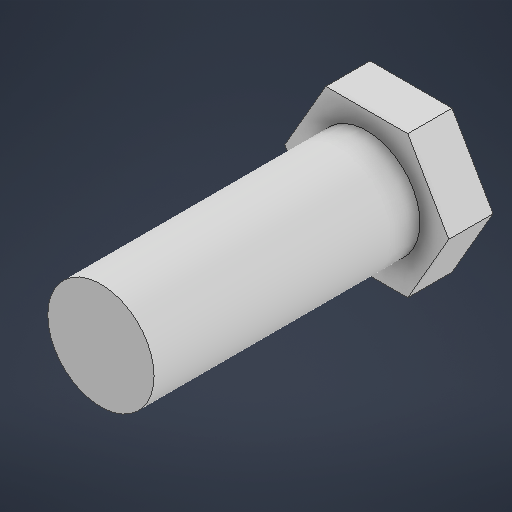
# Autodesk Inventor part: nut
Saved by Autodesk Inventor 2026 (Build 300175000, 175)
## iProperties
Created: 2025-05-07
Part Number: nut
Material: Generic
Document SubType Name: Modeling
Designer: Ritul Kumari
Density: 1 g/cm^3
Appearance: Default
Author: Ritul Kumari
Autodesk Inventor part; units mm, degrees
ref_plane "YZ Plane" through (0, 0, 0) normal (1, 0, 0) x (0, 1, 0)
ref_plane "XZ Plane" through (0, 0, 0) normal (0, 1, 0) x (-1, 0, 0)
ref_plane "XY Plane" through (0, 0, 0) normal (0, 0, 1) x (1, 0, 0)
sketch "Sketch1" plane through (0, 0, 0) normal (0, 0, 1) x (1, 0, 0)
  line L0 (1.6553, 0) -> (1.6553, 406.4)
  line L1 (562.1345, 203.2) -> (444.616, -0.348)
  line L2 (444.616, -0.348) -> (209.579, -0.348)
  line L3 (209.579, -0.348) -> (92.0605, 203.2)
  line L4 (92.0605, 203.2) -> (209.579, 406.748)
  line L5 (209.579, 406.748) -> (444.616, 406.748)
  line L6 (444.616, 406.748) -> (562.1345, 203.2)
  circle A0 centre (327.0975, 203.2) radius 152.4
  point P0 (0, 0)
  dimension "d0" = 406.4
  dimension "d1" = 304.8
  constraints: 14 end point, 1 centre point, 1 coincident, 1 vertical, 13 other
  measures "d0" distance of L0.start L0.end
  measures "d1" diameter of A0
extrude "Extrusion1" add sketch "Sketch1" along normal blind 127
sketch "Sketch2" plane through (0, 0, 127) normal (0, 0, 1) x (1, 0, 0)
  circle A0 centre (327.0975, 203.2) radius 152.4 projected
  circle A1 centre (327.0975, 203.2) radius 152.4
  point P0 (0, 0)
  dimension "d4" = 304.8
  constraints: 1 centre point, 1 coincident
  measures "d4" diameter of A1
extrude "Extrusion2" add sketch "Sketch2" along normal blind 762
body "Solid1"
